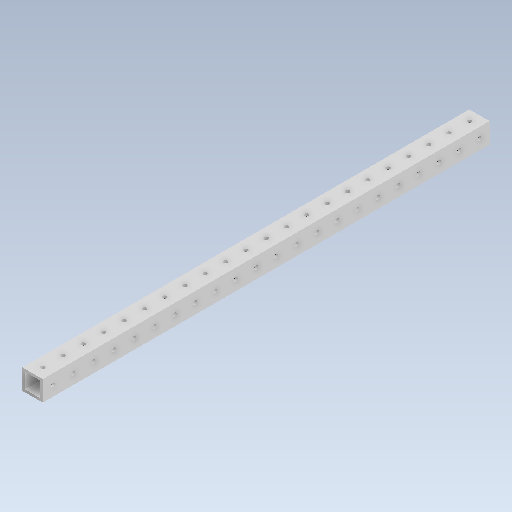
# Autodesk Inventor part: 1x1x18
Saved by Autodesk Inventor 2020 (Build 240168000, 168)
## iProperties
Created: 2020-01-19
Part Number: 1x1x18
Material: Generic
Document SubType Name: Modeling
Designer: srini
Density: 1 g/cm^3
Appearance: Default
Author: srini
Autodesk Inventor part; units mm, degrees
ref_plane "YZ Plane" through (0, 0, 0) normal (1, 0, 0) x (0, 1, 0)
ref_plane "XZ Plane" through (0, 0, 0) normal (0, 1, 0) x (-1, 0, 0)
ref_plane "XY Plane" through (0, 0, 0) normal (0, 0, 1) x (1, 0, 0)
sketch "Sketch1" plane through (0, 0, 0) normal (0, 0, 1) x (1, 0, 0)
  line L0 (-12.7, -12.7) -> (12.7, -12.7)
  line L1 (12.7, -12.7) -> (12.7, 12.7)
  line L2 (12.7, 12.7) -> (-12.7, 12.7)
  line L3 (-12.7, 12.7) -> (-12.7, -12.7)
  line L4 (-12.7, -12.7) -> (12.7, 12.7) construction
  line L5 (12.7, -12.7) -> (-12.7, 12.7) construction
  line L6 (-9.525, 9.525) -> (9.525, 9.525)
  line L7 (9.525, 9.525) -> (9.525, -9.525)
  line L8 (9.525, -9.525) -> (-9.525, -9.525)
  line L9 (-9.525, -9.525) -> (-9.525, 9.525)
  point P0 (0, 0)
  dimension "d0" = 25.4
  dimension "d1" = 25.4
  dimension "d2" = 3.175
  constraints: 20 end point, 4 parallel, 2 midpoint, 2 perpendicular, 1 horizontal, 3 other
  measures "d0" distance of L1.end L2.end
  measures "d1" distance of L0.end L1.end
  measures "d2" distance between parallel lines of L6 L2
extrude "Extrusion1" add sketch "Sketch1" along normal blind 558.8
sketch "Sketch2" plane through (-12.7, 12.7, 0) normal (0, 1, 0) x (1, 0, 0)
  circle A0 centre (12.7, -12.7) radius 2.54
  line L0 (0, 0) -> (0, -558.8) projected
  line L1 (25.4, 0) -> (0, 0) projected
  circle A1 centre (12.7, -38.1) radius 2.54
  circle A2 centre (12.7, -63.5) radius 2.54
  circle A3 centre (12.7, -88.9) radius 2.54
  circle A4 centre (12.7, -114.3) radius 2.54
  circle A5 centre (12.7, -139.7) radius 2.54
  circle A6 centre (12.7, -165.1) radius 2.54
  circle A7 centre (12.7, -190.5) radius 2.54
  circle A8 centre (12.7, -215.9) radius 2.54
  circle A9 centre (12.7, -241.3) radius 2.54
  circle A10 centre (12.7, -266.7) radius 2.54
  circle A11 centre (12.7, -292.1) radius 2.54
  circle A12 centre (12.7, -317.5) radius 2.54
  circle A13 centre (12.7, -342.9) radius 2.54
  circle A14 centre (12.7, -368.3) radius 2.54
  circle A15 centre (12.7, -393.7) radius 2.54
  circle A16 centre (12.7, -419.1) radius 2.54
  circle A17 centre (12.7, -444.5) radius 2.54
  circle A18 centre (12.7, -469.9) radius 2.54
  circle A19 centre (12.7, -495.3) radius 2.54
  circle A20 centre (12.7, -520.7) radius 2.54
  circle A21 centre (12.7, -546.1) radius 2.54
  point P0 (12.7, 0)
  dimension "d5" = 12.7
  dimension "d6" = 12.7
  dimension "d7" = 5.08
  dimension "d10" = 25.4
  constraints: 22 centre point, 1 vertical, 42 other
  measures "d5" distance from line of A0.centre L0
  measures "d6" distance from line of A0.centre L1
  measures "d7" diameter of A0
  measures "d10" distance of A0.centre A1.centre
extrude "Extrusion2" cut sketch "Sketch2" against normal through all
sketch "Sketch3" plane through (12.7, -12.7, 0) normal (1, 0, 0) x (0, 0, -1)
  circle A0 centre (-12.7, 12.7) radius 2.54
  line L0 (0, 0) -> (-558.8, 0) projected
  line L1 (0, 0) -> (0, 25.4) projected
  circle A1 centre (-38.1, 12.7) radius 2.54
  circle A2 centre (-63.5, 12.7) radius 2.54
  circle A3 centre (-88.9, 12.7) radius 2.54
  circle A4 centre (-114.3, 12.7) radius 2.54
  circle A5 centre (-139.7, 12.7) radius 2.54
  circle A6 centre (-165.1, 12.7) radius 2.54
  circle A7 centre (-190.5, 12.7) radius 2.54
  circle A8 centre (-215.9, 12.7) radius 2.54
  circle A9 centre (-241.3, 12.7) radius 2.54
  circle A10 centre (-266.7, 12.7) radius 2.54
  circle A11 centre (-292.1, 12.7) radius 2.54
  circle A12 centre (-317.5, 12.7) radius 2.54
  circle A13 centre (-342.9, 12.7) radius 2.54
  circle A14 centre (-368.3, 12.7) radius 2.54
  circle A15 centre (-393.7, 12.7) radius 2.54
  circle A16 centre (-419.1, 12.7) radius 2.54
  circle A17 centre (-444.5, 12.7) radius 2.54
  circle A18 centre (-469.9, 12.7) radius 2.54
  circle A19 centre (-495.3, 12.7) radius 2.54
  circle A20 centre (-520.7, 12.7) radius 2.54
  circle A21 centre (-546.1, 12.7) radius 2.54
  point P0 (0, 12.7)
  dimension "d17" = 12.7
  dimension "d18" = 12.7
  dimension "d19" = 5.08
  dimension "d22" = 25.4
  constraints: 22 centre point, 1 horizontal, 42 other
  measures "d17" distance from line of A0.centre L0
  measures "d18" distance from line of A0.centre L1
  measures "d19" diameter of A0
  measures "d22" distance of A0.centre A1.centre
extrude "Extrusion3" cut sketch "Sketch3" against normal through all
body "Solid1"
